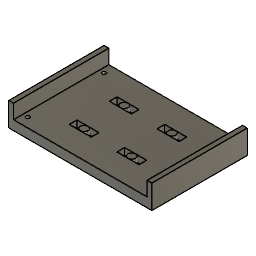
01_Spool_Roller_Base (Autodesk Fusion 360 design; units mm, degrees)
Autodesk Fusion 360 part; units mm, degrees
sketch "Sketch1" plane through (0, 0, 0) normal (0, 0, 1) x (1, 0, 0)
  line L0 (0, 0) -> (150, 0)
  line L1 (150, 0) -> (150, 100)
  line L2 (150, 100) -> (0, 100)
  line L3 (0, 100) -> (0, 0)
  dimension "d1" = 100
  dimension "d2" = 150
  constraint coincident L0.start L3.end
  measures "d1" distance of L0.start L2.end
  measures "d2" distance of L0.start L0.end
extrude "Extrude1" add sketch "Sketch1" along normal blind 10
sketch "Sketch2" plane through (0, 0, 10) normal (0, 0, 1) x (-1, 0, 0)
  line L0 (0, -100) -> (0, 0)
  line L1 (0, 0) -> (-150, 0)
  line L2 (-150, 0) -> (-150, -100)
  line L3 (-150, -100) -> (0, -100)
  line L4 (-38.5, -75) -> (-61.5, -75)
  line L5 (-61.5, -75) -> (-61.5, -67)
  line L6 (-61.5, -67) -> (-38.5, -67)
  line L7 (-38.5, -67) -> (-38.5, -75)
  line L8 (-111.5, -75) -> (-88.5, -75)
  line L9 (-88.5, -75) -> (-88.5, -67)
  line L10 (-88.5, -67) -> (-111.5, -67)
  line L11 (-111.5, -67) -> (-111.5, -75)
  dimension "d5" = 8
  dimension "d6" = 23
  dimension "d7" = 38.5
  dimension "d8" = 23
  dimension "d9" = 8
  dimension "d10" = 38.5
  dimension "d11" = 25
  dimension "d12" = 25
  constraint horizontal L4
  constraint vertical L5
  constraint horizontal L6
  constraint vertical L7
  constraint horizontal L8
  constraint vertical L9
  constraint horizontal L10
  constraint vertical L11
  measures "d5" distance of L4.end L5.end
  measures "d6" distance of L5.end L6.end
  measures "d7" distance of L0 L7
  measures "d8" distance of L9.end L10.end
  measures "d9" distance of L8.end L9.end
  measures "d10" distance of L2 L11
  measures "d11" distance of L3 L8
  measures "d12" distance of L3 L4
sketch "Sketch3" plane through (0, 0, 10) normal (0, 0, 1) x (-1, 0, 0)
  line L0 (-38.5, -25) -> (-61.5, -25)
  line L1 (-61.5, -25) -> (-61.5, -33)
  line L2 (-61.5, -33) -> (-38.5, -33)
  line L3 (-38.5, -33) -> (-38.5, -25)
  line L4 (0, -100) -> (0, 0)
  line L5 (0, 0) -> (-150, 0)
  line L6 (-111.5, -25) -> (-88.5, -25)
  line L7 (-88.5, -25) -> (-88.5, -33)
  line L8 (-88.5, -33) -> (-111.5, -33)
  line L9 (-111.5, -33) -> (-111.5, -25)
  line L10 (-150, 0) -> (-150, -100)
  dimension "d13" = 8
  dimension "d14" = 23
  dimension "d15" = 38.5
  dimension "d16" = 25
  dimension "d17" = 8
  dimension "d18" = 23
  dimension "d19" = 38.5
  dimension "d20" = 25
  constraint horizontal L0
  constraint vertical L1
  constraint horizontal L2
  constraint vertical L3
  constraint horizontal L6
  constraint vertical L7
  constraint horizontal L8
  constraint vertical L9
  measures "d13" distance of L0.end L1.end
  measures "d14" distance of L1.end L2.end
  measures "d15" distance of L3 L4
  measures "d16" distance of L0 L5
  measures "d17" distance of L6.end L7.end
  measures "d18" distance of L7.end L8.end
  measures "d19" distance of L9 L10
  measures "d20" distance of L5 L6
extrude "Extrude2" cut sketch "Sketch3" against normal blind 7
extrude "Extrude3" cut sketch "Sketch2" against normal blind 7 contours L4 L5 L6 L7 | L8 L9 L10 L11
sketch "Sketch4" plane through (0, 0, 3) normal (0, 0, 1) x (-1, 0, 0)
  line L0 (-38.5, -67) -> (-61.5, -67)
  line L1 (-61.5, -67) -> (-61.5, -75)
  line L2 (-61.5, -75) -> (-38.5, -75)
  line L3 (-38.5, -75) -> (-38.5, -67)
  line L4 (-38.5, -25) -> (-38.5, -33)
  circle A0 centre (-50, -29) radius 4
  line L5 (-61.5, -25) -> (-38.5, -25)
  line L6 (-61.5, -33) -> (-61.5, -25)
  circle A1 centre (-50, -71) radius 4
  circle A2 centre (-100, -71) radius 4
  line L7 (-111.5, -75) -> (-111.5, -67)
  line L8 (-88.5, -75) -> (-111.5, -75)
  circle A3 centre (-100, -29) radius 4
  line L9 (-111.5, -33) -> (-111.5, -25)
  line L10 (-88.5, -33) -> (-111.5, -33)
  dimension "d27" = 8
  dimension "d28" = 4
  dimension "d29" = 11.5
  dimension "d30" = 8
  dimension "d31" = 11.5
  dimension "d32" = 4
  dimension "d33" = 8
  dimension "d34" = 11.5
  dimension "d35" = 4
  dimension "d36" = 8
  dimension "d37" = 11.5
  dimension "d38" = 4
  measures "d27" diameter of A0
  measures "d28" distance of A0.centre L5
  measures "d29" distance of A0.centre L6
  measures "d30" diameter of A1
  measures "d31" distance of L3 A1.centre
  measures "d32" distance of L2 A1.centre
  measures "d33" diameter of A2
  measures "d34" distance of A2.centre L7
  measures "d35" distance of A2.centre L8
  measures "d36" diameter of A3
  measures "d37" distance of A3.centre L9
  measures "d38" distance of A3.centre L10
extrude "Extrude4" add sketch "Sketch4" along normal blind 7 contours A1 | A0 | A2 | A3
sketch "Sketch5" plane through (0, 0, 0) normal (0, 0, 1) x (1, 0, 0)
sketch "Sketch6" plane through (0, 0, 10) normal (0, 0, 1) x (-1, 0, 0)
  line L0 (-61.5, -75) -> (-61.5, -67)
  line L1 (-61.5, -67) -> (-50, -67)
  line L2 (-50, -67) -> (-38.5, -67)
  line L3 (-38.5, -67) -> (-38.5, -75)
  line L4 (-38.5, -75) -> (-50, -75)
  line L5 (-50, -75) -> (-61.5, -75)
  line L6 (-88.5, -75) -> (-100, -75)
  line L7 (-100, -75) -> (-111.5, -75)
  line L8 (-111.5, -75) -> (-111.5, -67)
  line L9 (-111.5, -67) -> (-100, -67)
  line L10 (-100, -67) -> (-88.5, -67)
  line L11 (-88.5, -67) -> (-88.5, -75)
  line L12 (-88.5, -25) -> (-88.5, -33)
  line L13 (-88.5, -33) -> (-100, -33)
  line L14 (-100, -33) -> (-111.5, -33)
  line L15 (-111.5, -33) -> (-111.5, -25)
  line L16 (-111.5, -25) -> (-100, -25)
  line L17 (-100, -25) -> (-88.5, -25)
  line L18 (-61.5, -25) -> (-50, -25)
  line L19 (-50, -25) -> (-38.5, -25)
  line L20 (-38.5, -25) -> (-38.5, -33)
  line L21 (-38.5, -33) -> (-50, -33)
  line L22 (-50, -33) -> (-61.5, -33)
  line L23 (-61.5, -33) -> (-61.5, -25)
  line L24 (0, -100) -> (0, 0)
  line L25 (0, 0) -> (-150, 0)
  line L26 (-150, 0) -> (-150, -100)
  line L27 (-150, -100) -> (0, -100)
  line L28 (0, -100) -> (-5, -100)
  line L29 (-5, -100) -> (-5, 0)
  line L30 (-5, 0) -> (0, 0)
  line L31 (0, 0) -> (0, -100)
  line L32 (-150, -100) -> (-145, -100)
  line L33 (-145, -100) -> (-145, 0)
  line L34 (-145, 0) -> (-150, 0)
  line L35 (-150, 0) -> (-150, -100)
  dimension "d42" = 5
  dimension "d43" = 100
  dimension "d44" = 5
  constraint horizontal L28
  constraint vertical L29
  constraint horizontal L30
  constraint vertical L31
  constraint coincident L25 L29.end
  constraint coincident L24.start L27.end
  constraint horizontal L32
  constraint vertical L33
  constraint horizontal L34
  constraint vertical L35
  constraint coincident L26.end L27.start
  measures "d42" distance of L29.end L24.end
  measures "d43" distance of L26.end L25.end
  measures "d44" distance of L26.end L32.end
extrude "Extrude5" add sketch "Sketch6" along normal blind 15 contours L24 L25 L27 L28 L29 L30 L31 | L25 L26 L27 L32 L33 L34 L35
sketch "Sketch7" plane through (0, 0, 10) normal (0, 0, 1) x (-1, 0, 0)
  line L0 (-145, 0) -> (-145, -100)
  line L1 (-145, -100) -> (-5, -100)
  line L2 (-5, -100) -> (-5, 0)
  line L3 (-5, 0) -> (-145, 0)
  line L4 (-61.5, -25) -> (-50, -25)
  line L5 (-50, -25) -> (-38.5, -25)
  line L6 (-38.5, -25) -> (-38.5, -33)
  line L7 (-38.5, -33) -> (-50, -33)
  line L8 (-50, -33) -> (-61.5, -33)
  line L9 (-61.5, -33) -> (-61.5, -25)
  line L10 (-88.5, -25) -> (-88.5, -33)
  line L11 (-88.5, -33) -> (-100, -33)
  line L12 (-100, -33) -> (-111.5, -33)
  line L13 (-111.5, -33) -> (-111.5, -25)
  line L14 (-111.5, -25) -> (-100, -25)
  line L15 (-100, -25) -> (-88.5, -25)
  line L16 (-88.5, -75) -> (-100, -75)
  line L17 (-100, -75) -> (-111.5, -75)
  line L18 (-111.5, -75) -> (-111.5, -67)
  line L19 (-111.5, -67) -> (-100, -67)
  line L20 (-100, -67) -> (-88.5, -67)
  line L21 (-88.5, -67) -> (-88.5, -75)
  line L22 (-61.5, -75) -> (-61.5, -67)
  line L23 (-61.5, -67) -> (-50, -67)
  line L24 (-50, -67) -> (-38.5, -67)
  line L25 (-38.5, -67) -> (-38.5, -75)
  line L26 (-38.5, -75) -> (-50, -75)
  line L27 (-50, -75) -> (-61.5, -75)
  circle A0 centre (-140, -10) radius 2
  circle A1 centre (-10, -10) radius 2
  circle A2 centre (-10, -90) radius 2
  circle A3 centre (-140, -90) radius 2
  line L28 (0, -100) -> (0, 0)
  line L29 (-150, 0) -> (-150, -100)
  dimension "d47" = 4
  dimension "d48" = 4
  dimension "d49" = 4
  dimension "d50" = 4
  dimension "d51" = 10
  dimension "d52" = 10
  dimension "d53" = 10
  dimension "d54" = 10
  dimension "d55" = 10
  dimension "d56" = 10
  dimension "d57" = 10
  dimension "d58" = 10
  measures "d47" diameter of A0
  measures "d48" diameter of A1
  measures "d49" diameter of A2
  measures "d50" diameter of A3
  measures "d51" distance of A1.centre L28
  measures "d52" distance of A0.centre L29
  measures "d53" distance of A3.centre L29
  measures "d54" distance of A2.centre L28
  measures "d55" distance of L1 A2.centre
  measures "d56" distance of L3 A1.centre
  measures "d57" distance of L3 A0.centre
  measures "d58" distance of L1 A3.centre
extrude "Extrude6" cut sketch "Sketch7" against normal blind 10 contours A0 | A1 | A2 | A3
